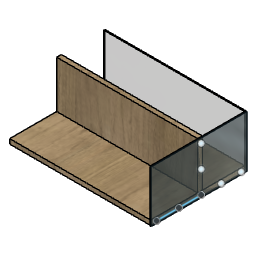
ionenantrieb v2 v1 (Autodesk Fusion 360 design; units mm, degrees)
Autodesk Fusion 360 part; units mm, degrees
sketch "Skizze1" plane through (0, 0, 0) normal (0, 0, 1) x (1, 0, 0)
  line L0 (0, 0) -> (300, 0)
  line L1 (300, 0) -> (300, 200)
  line L2 (300, 200) -> (0, 200)
  line L3 (0, 200) -> (0, 0)
  dimension "d1" = 300
  dimension "d2" = 200
  constraint horizontal L0
  constraint vertical L1
  constraint horizontal L2
  constraint vertical L3
  constraint coincident L0.start L3.end
  measures "d1" distance of L0.start L0.end
  measures "d2" distance of L0.start L2.end
extrude "Extrusion1" add sketch "Skizze1" along normal blind 10 makes body 1
sketch "Skizze2" plane through (0, 0, 10) normal (0, 0, 1) x (-1, 0, 0)
  line L0 (0, -200) -> (0, 0)
  line L1 (0, 0) -> (-300, 0)
  line L2 (-300, 0) -> (-300, -200)
  line L3 (-300, -200) -> (0, -200)
  line L4 (0, -100) -> (-300, -100)
  line L5 (-300, -100) -> (-300, -110)
  line L6 (-300, -110) -> (0, -110)
  line L7 (0, -110) -> (0, -100)
  constraint horizontal L4
  constraint vertical L5
  constraint horizontal L6
  constraint vertical L7
  constraint coincident L2 L5.end
  constraint midpoint L0 L4.start
extrude "Extrusion1'" add sketch "Skizze2" along normal blind 100 separate body contours L0 L2 L4 L5 L6 L7 makes body 2 in component "Component"
sketch "Skizze3" plane through (0, 200, 0) normal (0, 1, 0) x (-1, 0, 0)
  line L0 (-300, 0) -> (0, 0)
  line L1 (0, 0) -> (0, 10)
  line L2 (0, 10) -> (-300, 10)
  line L3 (-300, 10) -> (-300, 0)
  line L4 (-300, 0) -> (0, 0)
  line L5 (0, 0) -> (0, 110)
  line L6 (0, 110) -> (-300, 110)
  line L7 (-300, 110) -> (-300, 0)
  constraint horizontal L4
  constraint vertical L5
  constraint horizontal L6
  constraint vertical L7
  constraint coincident L0.start L3.end
extrude "Extrusion1''" add sketch "Skizze3" along normal blind 2.5 separate body makes body 3 in component "Component'"
sketch "Skizze4" plane through (0, 202.5, 0) normal (0, 1, 0) x (-1, 0, 0)
  line L0 (-300, 110) -> (-300, 0)
  line L1 (-300, 0) -> (0, 0)
  line L2 (0, 0) -> (0, 110)
  line L3 (0, 110) -> (-300, 110)
  circle A0 centre (-290, 5) radius 1
  circle A1 centre (-220, 5) radius 1
  circle A2 centre (-150, 5) radius 1
  circle A3 centre (-80, 5) radius 1
  circle A4 centre (-10, 5) radius 1
  dimension "d9" = 2
  dimension "d12" = 280
  dimension "d13" = 0
  measures "d9" diameter of A0
extrude "Extrusion2" cut sketch "Skizze4" against normal blind 2.5 contours A0 | A1 | A2 | A3 | A4 bodies 3 in component "Component'"
sketch "Skizze5" plane through (300, 0, 0) normal (1, 0, 0) x (0, 1, 0)
  line L0 (0, 0) -> (200, 0)
  line L1 (200, 0) -> (200, 10)
  line L2 (200, 10) -> (0, 10)
  line L3 (0, 10) -> (0, 0)
  line L4 (202.5, 0) -> (-1.5, 0)
  line L5 (-1.5, 0) -> (-1.5, 110)
  line L6 (-1.5, 110) -> (202.5, 110)
  line L7 (202.5, 110) -> (202.5, 0)
  dimension "d16" = 204
  constraint horizontal L4
  constraint vertical L5
  constraint horizontal L6
  constraint vertical L7
  measures "d16" distance of L4.start L4.end
extrude "Extrusion1'''" add sketch "Skizze5" along normal blind 2.5 separate body makes body 4 in component "Component''"
sketch "Skizze6" plane through (302.5, 0, 0) normal (1, 0, 0) x (0, 1, 0)
  line L0 (202.5, 110) -> (-1.5, 110)
  line L1 (-1.5, 110) -> (-1.5, 0)
  line L2 (-1.5, 0) -> (202.5, 0)
  line L3 (202.5, 0) -> (202.5, 110)
  circle A0 centre (10, 5) radius 1
  circle A1 centre (105, 5) radius 1
  line L4 (10, 5) -> (105, 5)
  circle A2 centre (57.5, 5) radius 1
  circle A3 centre (147.5, 5) radius 1
  circle A4 centre (190, 5) radius 1
  circle A5 centre (105, 52.5) radius 1
  circle A6 centre (105, 100) radius 1
  dimension "d19" = 2
  dimension "d20" = 2
  dimension "d21" = 2
  dimension "d24" = 85
  dimension "d25" = 0
  dimension "d28" = 0
  dimension "d29" = 95
  constraint coincident A0.centre L4.start
  constraint coincident A1.centre L4.end
  constraint midpoint L4 A2.centre
  measures "d19" diameter of A0
  measures "d20" diameter of A1
  measures "d21" diameter of A2
component "Component" placed x (1, 0, 0) y (0, 1, 0) z (0, 0, 1) at (0, 0, 0)
component "Component'" placed x (1, 0, 0) y (0, 1, 0) z (0, 0, 1) at (0, 0, 0)
component "Component''" placed x (1, 0, 0) y (0, 1, 0) z (0, 0, 1) at (0, 0, 0)
